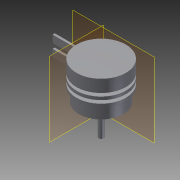
# Autodesk Inventor part: BallHolder
Saved by Autodesk Inventor 2012 (Build 160160000, 160)
## iProperties
Created: 2013-07-08
Part Number: BallHolder
Material: Default
Document SubType Name: Modeling
Designer: 1
Density: 1 g/cm^3
Author: 1
Autodesk Inventor part; units mm, degrees
ref_plane "XZ Plane" through (0, 0, 0) normal (0, 1, 0) x (-1, 0, 0)
sketch "Sketch1" plane through (0, 0, 0) normal (0, 0, 1) x (1, 0, 0)
  line L0 (-18, 0) -> (-18, 10)
  line L1 (-18, 10) -> (-20, 10)
  line L2 (-20, 10) -> (-20, 12.5)
  line L3 (-20, 12.5) -> (-15, 12.5)
  line L4 (-15, 12.5) -> (-15, 15)
  line L5 (-15, 15) -> (-20, 15)
  line L6 (-20, 15) -> (-20, 17.5)
  line L7 (-20, 17.5) -> (-15, 17.5)
  line L8 (-15, 17.5) -> (-15, 20)
  line L9 (-15, 20) -> (-20, 20)
  line L10 (-20, 20) -> (-20, 30)
  line L11 (-20, 30) -> (0, 30)
  line L12 (0, 30) -> (0, 0)
  line L13 (-18, 0) -> (-12, 0)
  line L14 (-12, 5) -> (-2, 5)
  line L15 (-12, 0) -> (-18, 0)
  line L16 (-2, -25) -> (0, -25)
  line L17 (0, 0) -> (0, -25)
  line L18 (-2, 5) -> (-2, -25)
  line L19 (-12, 5) -> (-12, 0)
  dimension "d0" = 2.5
  dimension "d1" = 20
  dimension "d3" = 5
  dimension "d4" = 10
  dimension "d22" = 10
  dimension "d24" = 30
  dimension "d26" = 2
  dimension "d27" = 25
  dimension "d28" = 10
  dimension "d29" = 30
  dimension "d30" = 18
  constraints: 40 end point, 8 parallel, 7 perpendicular, 3 collinear, 3 equal length, 1 point on line, 1 vertical
  measures "d0" distance of L5.end L6.end
  measures "d1" distance of L10.end L11.end
  measures "d3" distance between parallel lines of L10 L8
  measures "d4" distance between parallel lines of L11 L9
  measures "d22" distance of L14.start L14.end
  measures "d24" distance between parallel lines of L14 L16
  measures "d26" distance of L16.start L16.end
  measures "d27" distance between parallel lines of L14 L11
  measures "d28" distance between parallel lines of L13 L1
  measures "d29" distance from line of point (0, 0) L11
  measures "d30" distance between parallel lines of L12 L0
revolve "Revolution1" add sketch "Sketch1" angle 360 about axis through (0, 30, 0) along (0, -1, 0)
ref_plane "Work Plane4" through (-20, 16.25, 0) normal (1, 0, 0) x (0, 1, 0)
sketch "Sketch6" plane through (-20, 16.25, 0) normal (1, 0, 0) x (0, 1, 0)
  line L0 (4.3754, -2.422) -> (10.3754, -2.422)
  line L1 (10.3754, -2.422) -> (10.3754, -0.6353)
  line L2 (10.3754, -0.6353) -> (4.3754, -0.6353)
  line L3 (4.3754, -0.6353) -> (4.3754, -2.422)
  line L4 (0.3754, -0.6353) -> (-5.6246, -0.6353)
  line L5 (-5.6246, -0.6353) -> (-5.6246, -2.422)
  line L6 (-5.6246, -2.422) -> (0.3754, -2.422)
  line L7 (0.3754, -2.422) -> (0.3754, -0.6353)
  line L8 (-830.9186, 0) -> (19.0814, 0) projected
  point P0 (0, 0)
  dimension "d39" = 6
  dimension "d40" = 6
  dimension "d41" = 10
  dimension "d42" = 1.7867
  dimension "d43" = 1.7867
  dimension "d44" = 10.3753
  dimension "d45" = 0.6353
  dimension "d46" = 0.6353
  dimension "d47" = 8.706
  constraints: 16 end point, 4 parallel, 2 horizontal, 2 perpendicular, 1 point on line
  measures "d39" distance of L5.end L6.end
  measures "d40" distance of L0.start L0.end
  measures "d41" distance between parallel lines of L1 L7
  measures "d42" distance between parallel lines of L0 L2
  measures "d43" distance between parallel lines of L2 L6
  measures "d44" distance from line of point (0, 0) L1
  measures "d45" distance from line of point (0, 0) L2
  measures "d46" distance between parallel lines of L8 L2
  measures "d47" distance from line of L8.end L1
extrude "Extrusion2" add sketch "Sketch6" along normal blind 21.1125 and the other way blind 20.081
ref_plane "Work Plane5" through (0, 25, -20) normal (0, 0, 1) x (1, 0, 0)
sketch "Sketch7" plane through (0, 25, -20) normal (0, 0, 1) x (1, 0, 0)
  circle A0 centre (0, -20) radius 2.5
  point P0 (0, -25)
  dimension "d48" = 5
  dimension "d49" = 5
  constraints: 1 centre point
  measures "d48" diameter of A0
  measures "d49" distance of A0.centre point (0, -25)
extrude "Extrusion3" add sketch "Sketch7" along normal blind 36.4625 and the other way blind 3.944
body "Solid1"
